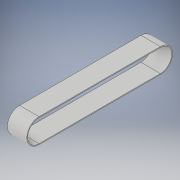
# Autodesk Inventor part: nhk6
Saved by Autodesk Inventor 2019 (Build 230136000, 136)
## iProperties
Created: 2022-02-10
Part Number: nhk6
Material: 一般
Document SubType Name: Sheet Metal
Designer: yuta
Density: 1 g/cm^3
Sheet Metal Rule: Default_mm
Appearance: 既定
Author: yuta
Autodesk Inventor part; units mm, degrees
ref_plane "YZ Plane" through (0, 0, 0) normal (1, 0, 0) x (0, 1, 0)
ref_plane "XZ Plane" through (0, 0, 0) normal (0, 1, 0) x (-1, 0, 0)
ref_plane "XY Plane" through (0, 0, 0) normal (0, 0, 1) x (1, 0, 0)
sketch "スケッチ1" plane through (0, 0, 0) normal (1, 0, 0) x (0, 1, 0)
  line L0 (-44.8898, -5.203) -> (-44.8898, -255.203)
  line L1 (5.1102, -255.203) -> (5.1102, -5.203)
  arc A0 (5.1102, -5.203) -> (-44.8898, -5.203) centre (-19.8898, -5.203) ccw
  arc A1 (-44.8898, -255.203) -> (5.1102, -255.203) centre (-19.8898, -255.203) ccw
  point P0 (0, 0)
  dimension "d2" = 50
  dimension "d3" = 50
  dimension "d4" = 250
  dimension "d5" = 250
  dimension "d6" = 50
  dimension "d7" = 50
  constraints: 4 end point, 4 point on circle, 2 centre point, 1 parallel
  measures "d2" diameter of A0
  measures "d3" diameter of A1
  measures "d4" distance of L1.start L1.end
  measures "d5" distance of L0.start L0.end
  measures "d6" distance of L0.start L1.end
  measures "d7" distance between parallel lines of L0 L1
extrude "押し出し1" add sketch "スケッチ1" along normal blind 40
sketch "スケッチ2" plane through (40, 0, 0) normal (1, 0, 0) x (0, 0, -1)
  line L0 (5.203, 3.2402) -> (255.203, 3.2402)
  line L1 (255.203, -43.0198) -> (5.203, -43.0198)
  line L2 (5.203, -44.8898) -> (255.203, -44.8898) projected
  arc A0 (5.203, 5.1102) -> (5.203, -44.8898) centre (5.203, -19.8898) ccw projected
  arc A1 (5.203, 3.2402) -> (5.203, -43.0198) centre (5.203, -19.8898) ccw
  arc A2 (255.203, -43.0198) -> (255.203, 3.2402) centre (255.203, -19.8898) ccw
  line L3 (255.203, 3.2402) -> (255.203, 3.2402)
  line L4 (255.203, -43.0198) -> (255.203, -43.0198)
  point P0 (0, 0)
  dimension "d12" = 1.87
  dimension "d14" = 46.26
  dimension "d15" = 46.26
  dimension "d16" = 250
  dimension "d17" = 46.26
  dimension "d18" = 250
  constraints: 8 end point, 6 point on circle, 2 centre point, 2 perpendicular, 1 horizontal, 1 parallel
  measures "d12" distance between parallel lines of L1 L2
  measures "d14" diameter of A1
  measures "d15" diameter of A2
  measures "d16" distance of L1.start L1.end
  measures "d17" distance between parallel lines of L0 L1
  measures "d18" distance of L0.end L0.start
extrude "押し出し2" cut sketch "スケッチ2" against normal blind 40
equation "\"BendRadius\" = Thickness"
equation "\"BendReliefWidth\" = Thickness"
equation "\"BendReliefDepth\" = 0.5 * Thickness"
equation "\"CornerReliefSize\" = 4 * Thickness"
equation "\"MinimumRemnant\" = 2 * Thickness"
equation "\"TransitionRadius\" = BendRadius"
equation "\"JacobiRadiusSize\" = BendRadius"
equation "\"GapSize\" = Thickness"
equation "\"Thickness\" = 0.5"
